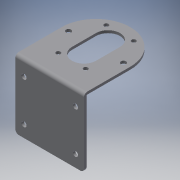
# Autodesk Inventor part: MotorMount
Saved by Autodesk Inventor 2018 (Build 220112000, 112)
## iProperties
Created: 2021-04-30
Part Number: MotorMount
Material: Generic
Document SubType Name: Modeling
Designer: dangl
Density: 1 g/cm^3
Appearance: Default
Author: dangl
Autodesk Inventor part; units mm, degrees
ref_plane "YZ Plane" through (0, 0, 0) normal (1, 0, 0) x (0, 1, 0)
ref_plane "XZ Plane" through (0, 0, 0) normal (0, 1, 0) x (-1, 0, 0)
ref_plane "XY Plane" through (0, 0, 0) normal (0, 0, 1) x (1, 0, 0)
sketch "Sketch1" plane through (0, 0, 0) normal (1, 0, 0) x (0, 1, 0)
  line L0 (0, 0) -> (38, 0)
  line L1 (40, -2) -> (40, -47)
  arc A0 (40, -2) -> (38, 0) centre (38, -2) ccw
  line L2 (38.5, -47) -> (38.5, -2)
  arc A1 (38.5, -2) -> (38, -1.5) centre (38, -2) ccw
  line L3 (38, -1.5) -> (0, -1.5)
  line L4 (40, -47) -> (38.5, -47)
  line L5 (0, 0) -> (0, -1.5)
  point P0 (40, 0)
  dimension "d0" = 47
  dimension "d1" = 40
  dimension "d2" = 2
  dimension "d3" = 1.5
  constraints: 12 end point, 4 point on circle, 2 centre point, 2 horizontal, 2 point on line, 2 tangent, 1 perpendicular, 1 vertical, 2 other
  measures "d0" distance of point (40, 0) L1.end
  measures "d1" distance of L0.start point (40, 0)
  measures "d2" radius of A0
  measures "d3" distance between parallel lines of L1 L2
extrude "Extrusion1" add sketch "Sketch1" along normal mid plane 40
fillet "Fillet1" radius 20 2 edges at (20, 39.25, -47) (-20, 39.25, -47)
fillet "Fillet2" radius 2 2 edges at (-20, 0, -0.75) (20, 0, -0.75)
sketch "Sketch2" plane through (-20, 38, 0) normal (0, 0, 1) x (1, 0, 0)
  circle A0 centre (5, -7) radius 1.5 projected
  circle A1 centre (5, -31) radius 1.5 projected
  circle A2 centre (35, -31) radius 1.5 projected
  circle A3 centre (35, -7) radius 1.5 projected
  point P0 (20, -38)
extrude "Extrusion2" cut sketch "Sketch2" against normal through all
sketch "Sketch3" plane through (-20, 40, -2) normal (0, 1, 0) x (1, 0, 0)
  arc A0 (13, 18) -> (27, 18) centre (20, 18) ccw
  arc A1 (27, 32) -> (13, 32) centre (20, 32) ccw
  line L0 (13, 18) -> (13, 32)
  line L1 (27, 18) -> (27, 32)
  arc A2 (40, 25) -> (0, 25) centre (20, 25) ccw projected
  circle A3 centre (36, 25) radius 1.5
  circle A4 centre (4, 25) radius 1.5
  circle A5 centre (28, 11) radius 1.25
  circle A6 centre (12, 11) radius 1.25
  line L2 (40, 0) -> (40, 25) projected
  line L3 (40, 25) -> (0, 25)
  circle A7 centre (28, 39) radius 1.25
  circle A8 centre (12, 39) radius 1.25
  point P0 (20, -2)
  dimension "d10" = 14
  dimension "d11" = 14
  dimension "d12" = 28
  dimension "d13" = 7
  dimension "d14" = 3
  dimension "d15" = 3
  dimension "d16" = 32
  dimension "d17" = 16
  dimension "d18" = 2.5
  dimension "d19" = 2.5
  dimension "d20" = 16
  dimension "d21" = 8
  constraints: 8 centre point, 6 end point, 4 point on circle, 2 symmetric about line, 2 tangent, 1 parallel, 1 perpendicular, 1 vertical, 2 other
  measures "d10" diameter of A0
  measures "d11" diameter of A1
  measures "d13" distance of A2.centre A1.centre
  measures "d14" diameter of A3
  measures "d15" diameter of A4
  measures "d16" distance of A4.centre A3.centre
  measures "d17" distance of A2.centre A3.centre
  measures "d18" diameter of A5
  measures "d19" diameter of A6
  measures "d20" distance of A6.centre A5.centre
  measures "d21" horizontal distance of A0.centre A6.centre
extrude "Extrusion3" cut sketch "Sketch3" against normal through all contours L0 L3 L1 A0 | L0 A1 L1 L3 | L3 A4 | A4 L3 | L3 A3 | A3 L3 | A5 | A6 | A7 | A8
equation "\"d17\" = 0.5 * d16"
equation "\"d21\" = 0.5 * d20"
body "Solid1"
